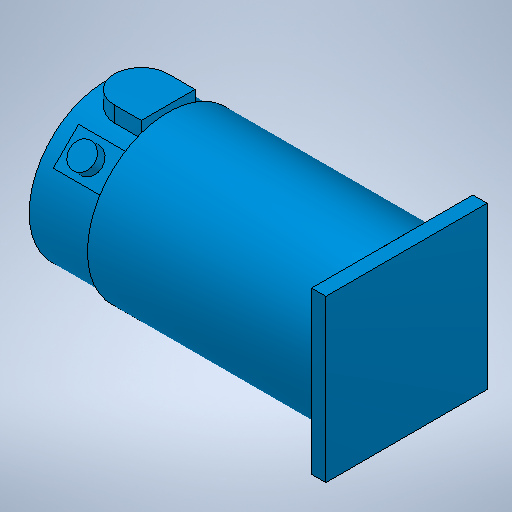
# Autodesk Inventor part: temporary_motor
Saved by Autodesk Inventor 2025.3 (Build 293356030, 356C)
## iProperties
Created: 2025-08-09
Part Number: temporary_motor
Material: 알루미늄 6061
Document SubType Name: Modeling
Designer: LeeJinWon
Density: 3.17401 g/cm^3
Appearance: 알루미늄 - 평지
Project: Robot Arm
Mass: 3400 g
Surface Area: 655.166 cm^2
Volume: 1071.2 cm^3
Author: LeeJinWon
Autodesk Inventor part; units mm, degrees
ref_plane "YZ Plane" through (0, 0, 0) normal (1, 0, 0) x (0, 1, 0)
sketch "스케치1" plane through (0, 0, 0) normal (1, 0, 0) x (0, 1, 0)
  circle A0 centre (0, 0) radius 45
  dimension "d0" = 90
  constraints: 1 centre point, 1 coincident
  measures "d0" diameter of A0
extrude "돌출1" add sketch "스케치1" along normal mid plane 160
sketch "스케치2" plane through (80, 0, 0) normal (1, 0, 0) x (0, 0, -1)
  line L0 (-45, 45) -> (45, 45)
  line L1 (45, 45) -> (45, -45)
  line L2 (45, -45) -> (-45, -45)
  line L3 (-45, -45) -> (-45, 45)
  line L4 (-45, 45) -> (45, -45) construction
  line L5 (45, 45) -> (-45, -45) construction
  circle A0 centre (0, 0) radius 45 projected
  point P0 (0, 0)
  constraints: 12 end point, 3 tangent, 2 midpoint, 2 parallel, 2 perpendicular, 1 horizontal
extrude "돌출2" add sketch "스케치2" along normal blind 8
sketch "스케치4" plane through (-80, 0, 0) normal (-1, 0, 0) x (0, 0, 1)
  circle A0 centre (0, 0) radius 42.5
  circle A1 centre (0, 0) radius 45 projected
  dimension "d15" = 85
  constraints: 1 centre point, 1 coincident
  measures "d15" diameter of A0
extrude "돌출3" cut sketch "스케치4" against normal blind 35
ref_plane "작업 평면1" through (-80, 42.5, 0) normal (0, 1, 0) x (-1, 0, 0)
sketch "스케치5" plane through (-80, 42.5, 0) normal (0, 1, 0) x (-1, 0, 0)
  line L0 (-35, -42.5) -> (-35, 42.5) projected
  line L1 (-35, -15) -> (-20, -15)
  line L2 (-20, -15) -> (-20, 15)
  line L3 (-20, 15) -> (-35, 15)
  line L4 (-35, 15) -> (-35, -15)
  circle A0 centre (-20, 0) radius 15
  point P0 (-80, 0)
  point P1 (-35, 0)
  point P2 (-35, 0)
  point P3 (-20, -15)
  dimension "d18" = 30
  dimension "d25" = 30
  constraints: 8 end point, 3 midpoint, 2 parallel, 1 coincident, 1 horizontal, 1 perpendicular, 1 point on line, 3 other
  measures "d18" distance of L1.end L2.end
extrude "돌출4" add sketch "스케치5" along normal mid plane 12
sketch "스케치3" plane through (88, 0, 0) normal (1, 0, 0) x (0, 0, -1)
  line L0 (-36.5, 36.5) -> (36.5, 36.5) construction
  line L1 (36.5, 36.5) -> (36.5, -36.5) construction
  line L2 (36.5, -36.5) -> (-36.5, -36.5) construction
  line L3 (-36.5, -36.5) -> (-36.5, 36.5) construction
  line L4 (-36.5, 36.5) -> (36.5, -36.5) construction
  line L5 (36.5, 36.5) -> (-36.5, -36.5) construction
  point P0 (0, 0)
  dimension "d6" = 73
  dimension "d7" = 73
  constraints: 12 end point, 2 midpoint, 2 parallel, 1 horizontal, 1 perpendicular
  measures "d6" distance of L1.end L2.end
  measures "d7" distance of L0.end L1.end
mirror "미러1" about plane through (0, 0, 0) normal (0, 1, 0) of "돌출4"
sketch "스케치6" plane through (-80, 0, 0) normal (-1, 0, 0) x (0, 0, 1)
  line L0 (0, 0) -> (30.052, 30.052) construction
  circle A0 centre (0, 0) radius 42.5 projected
  line L1 (42.5, 0) -> (0, 0) construction
  dimension "d21" = 45
  constraints: 4 end point, 2 point on circle, 1 horizontal
  measures "d21" angle of L0 L1
ref_plane "작업 평면2" through (-80, 30.052, 30.052) normal (0, 0.7071068, 0.7071068) x (-1, 0, 0)
sketch "스케치7" plane through (-80, 30.052, 30.052) normal (0, 0.7071068, 0.7071068) x (-1, 0, 0)
  line L0 (-8.7137, -10) -> (-38.7137, -10)
  line L1 (-38.7137, -10) -> (-38.7137, 10)
  line L2 (-38.7137, 10) -> (-8.7137, 10)
  line L3 (-8.7137, 10) -> (-8.7137, -10)
  point P0 (-80, 0)
  point P1 (0, 0)
  point P2 (-8.7137, 0)
  dimension "d22" = 20
  dimension "d26" = 30
  constraints: 8 end point, 2 parallel, 1 horizontal, 1 horizontal alignment, 1 midpoint, 1 perpendicular
  measures "d22" distance of L2.end L0.start
  measures "d26" distance between parallel lines of L1 L3
extrude "돌출5" add sketch "스케치7" along normal mid plane 2
sketch "스케치8" plane through (-80, 30.7591, 30.7591) normal (0, 0.7071068, 0.7071068) x (1, 0, 0)
  circle A0 centre (22, 0) radius 7
  line L0 (8.7137, 10) -> (8.7137, -10) projected
  line L1 (35, -45) -> (35, 19.3934) projected
  point P0 (80, 0)
  point P1 (8.7137, 0)
  point P2 (35, -40.6066)
  dimension "d27" = 14
  dimension "d29" = 20
  constraints: 1 centre point, 1 horizontal alignment, 1 midpoint
  measures "d27" diameter of A0
extrude "돌출6" add sketch "스케치8" along normal blind 6
